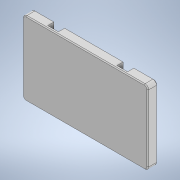
# Autodesk Inventor part: BatteryHolder
Saved by Autodesk Inventor 2022 (Build 260153000, 153)
## iProperties
Created: 2021-11-25
Part Number: BatteryHolder
Material: Generic
Document SubType Name: Modeling
Designer: Viktor
Density: 1 g/cm^3
Appearance: Default
Author: Viktor
## iProperties of the stored document BatteryHolder_3DPrint.ipt
Created: 2021-11-25
Part Number: BatteryHolder_3DPrint
Material: Generic
Document SubType Name: Modeling
Designer: Viktor
Density: 1 g/cm^3
Appearance: Default
Author: Viktor
Autodesk Inventor part; units mm, degrees
ref_plane "YZ Plane" through (0, 0, 0) normal (1, 0, 0) x (0, 1, 0)
ref_plane "XZ Plane" through (0, 0, 0) normal (0, 1, 0) x (-1, 0, 0)
ref_plane "XY Plane" through (0, 0, 0) normal (0, 0, 1) x (1, 0, 0)
sketch "Sketch1" plane through (0, 0, 0) normal (0, 0, 1) x (1, 0, 0)
  line L0 (-52.5, -31) -> (52.5, -31)
  line L1 (52.5, -31) -> (52.5, 31)
  line L2 (52.5, 31) -> (-52.5, 31)
  line L3 (-52.5, 31) -> (-52.5, -31)
  line L4 (-52.5, -31) -> (52.5, 31) construction
  line L5 (52.5, -31) -> (-52.5, 31) construction
  point P0 (0, 0)
  dimension "d1" = 105
  dimension "d2" = 62
  constraints: 12 end point, 2 midpoint, 2 parallel, 1 horizontal, 1 perpendicular
  measures "d1" distance between parallel lines of L1 L3
  measures "d2" distance between parallel lines of L0 L2
extrude "Extrusion1" add sketch "Sketch1" along normal blind 8
sketch "Sketch2" plane through (0, 0, 0) normal (0, 0, -1) x (-1, 0, 0)
  line L0 (-52.5, -31) -> (-52.5, 31) projected
  line L1 (52.5, -31) -> (-52.5, -31) projected
  line L2 (52.5, 31) -> (52.5, -31) projected
  line L3 (-52.5, 31) -> (52.5, 31) projected
  line L4 (52.5, -31) -> (-52.5, -31) projected
  line L5 (33.5, -31) -> (24.5, -31)
  line L6 (24.5, -31) -> (24.5, 31)
  line L7 (24.5, 31) -> (33.5, 31)
  line L8 (33.5, 31) -> (33.5, -31)
  line L9 (-73.5, 0) -> (73.5, 0) construction
  line L10 (0, -43.4) -> (0, 43.4) construction
  line L11 (-33.5, -31) -> (-24.5, -31)
  line L12 (-24.5, -31) -> (-24.5, 31)
  line L13 (-24.5, 31) -> (-33.5, 31)
  line L14 (-33.5, 31) -> (-33.5, -31)
  point P0 (0, 0)
  point P1 (-33.5, 31)
  point P2 (-24.5, 31)
  point P3 (33.5, 31)
  dimension "d5" = 9
  dimension "d6" = 19
  constraints: 16 end point, 4 symmetric about line, 2 parallel, 2 point on line, 1 horizontal, 1 perpendicular
  measures "d5" distance between parallel lines of L6 L8
  measures "d6" distance between parallel lines of L2 L8
extrude "Extrusion2" cut sketch "Sketch2" against normal blind 4 contours L14 L3 L12 L1 | L6 L3 L8 L1
chamfer "Chamfer1" distance 2 angle 45 4 edges at (-29, -31, 4) (29, -31, 4) (29, 31, 4) (-29, 31, 4)
fillet "Fillet1" radius 3 4 edges at (-52.5, -31, 4) (-52.5, 31, 4) (52.5, -31, 4) (52.5, 31, 4)
chamfer "Chamfer2" distance 0.75 angle 45 4 edges at (0, -31, 8) (-52.5, 0, 8) (0, 31, 8) (52.5, 0, 8)
chamfer "Chamfer3" distance 0.75 angle 45 16 edges at (-52.5, 0, 0) (-51.6213, -30.1213, 0) (-41.5, -31, 0) (-51.6213, 30.1213, 0) (-41.5, 31, 0) (52.5, 0, 0) (51.6213, 30.1213, 0) (41.5, 31, 0) (51.6213, -30.1213, 0) (41.5, -31, 0) (0, 31, 0) (24.5, 0, 0) (0, -31, 0) (-24.5, 0, 0) (-33.5, 0, 0) (33.5, 0, 0)
body "Solid1"
